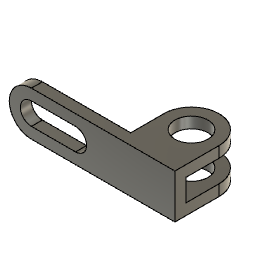
Model 10 (Autodesk Fusion 360 design; units mm, degrees)
Autodesk Fusion 360 part; units mm, degrees
sketch "Sketch4" plane through (0, 0, 0) normal (0, 1, 0) x (1, 0, 0)
  line L0 (0, 0) -> (130, 0)
  line L1 (130, 0) -> (130, -40)
  line L2 (130, -40) -> (0, -40)
  line L3 (130, -40) -> (130, -30)
  line L4 (130, -40) -> (130, -30)
  line L5 (130, -30) -> (80, -30)
  line L6 (80, -30) -> (80, -40)
  line L7 (130, 0) -> (130, -10)
  line L8 (130, -10) -> (80, -10)
  line L9 (80, -10) -> (80, 0)
  arc A0 (0, 0) -> (0, -40) centre (0, -20) ccw
  line L10 (0, -20) -> (40, -20) construction
  line L11 (0, -20) -> (0, -30) construction
  line L12 (40, -20) -> (40, -30) construction
  line L13 (40, -30) -> (0, -30)
  line L14 (0, -20) -> (0, -10) construction
  line L15 (0, -10) -> (40, -10)
  arc A1 (0.0017, -10) -> (0, -30) centre (0, -20) ccw
  arc A2 (40, -30) -> (40, -10) centre (40, -20) ccw
  dimension "d16" = 130
  dimension "d17" = 40
  dimension "d18" = 10
  dimension "d19" = 50
  dimension "d20" = 10
  dimension "d21" = 50
  dimension "d22" = 20
  dimension "d23" = 40
  dimension "d24" = 40
  dimension "d25" = 20
  constraint horizontal L0
  constraint vertical L1
  constraint horizontal L2
  constraint coincident L0.start A0.start
  constraint coincident L1 L3.end
  constraint perpendicular L2 L4
  constraint perpendicular L4 L5
  constraint coincident L2 L6.end
  constraint perpendicular L2 L6
  constraint coincident L1 L7.end
  constraint perpendicular L1 L8
  constraint coincident L0 L9.end
  constraint perpendicular L0 L9
  constraint concentric A0 A1
  constraint coincident A0.centre L10.start
  constraint parallel L5 L10
  constraint coincident L10.end L12.start
  constraint perpendicular L10 L11
  constraint perpendicular L10 L12
  constraint coincident L14.end A1
  constraint perpendicular L10 L14
  constraint tangent L15 A2
  constraint coincident L15 A1.start
  measures "d16" distance of L0.start L0.end
  measures "d17" distance of L0.start L2.end
  measures "d18" distance of L1.end L3.end
  measures "d19" distance of L3.end L5.end
  measures "d20" distance of L0.end L7.end
  measures "d21" distance of L7.end L8.end
  measures "d22" diameter of A1
  measures "d23" diameter of A0
  measures "d24" distance of A0.centre L10.end
  measures "d25" diameter of A2
extrude "Extrude5" add sketch "Sketch4" along normal blind 10 contours L0 L1 L2 L5 L6 L8 L9 A0
extrude "Extrude6" add sketch "Sketch4" along normal blind 75 contours L0 L1 L7 L8 L9 | L1 L2 L3 L4 L5 L6
sketch "Sketch5" plane through (0, 0, 40) normal (0, 0, 1) x (-1, 0, 0)
  line L0 (0, 0) -> (-130, 0)
  line L1 (-130, 0) -> (-130, -75)
  line L2 (-130, -75) -> (-80, -75)
  line L3 (-80, -75) -> (-80, -10)
  line L4 (-80, -10) -> (0, -10)
  line L5 (0, -10) -> (0, 0)
  line L6 (-130, 0) -> (-130, -40) construction
  line L7 (-130, -40) -> (-80, -40) construction
  circle A0 centre (-105, -40) radius 15
  arc A1 (-130, -40) -> (-80, -40) centre (-105, -40) ccw
  dimension "d30" = 40
  dimension "d31" = 30
  dimension "d32" = 50
  constraint coincident L0.end L1.start
  constraint perpendicular L0 L6
  constraint coincident L3 L7.end
  constraint perpendicular L3 L7
  constraint midpoint L7 A0.centre
  constraint concentric A0 A1
  measures "d30" distance of L0.end L6.end
  measures "d31" diameter of A0
  measures "d32" diameter of A1
extrude "Extrude7" cut sketch "Sketch5" against normal blind 40 contours L1 L2 L3 A1
extrude "Extrude8" cut sketch "Sketch5" against normal blind 40 contours A0
